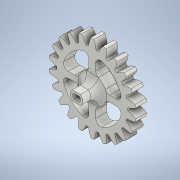
# Autodesk Inventor part: Spur Gear111
Saved by Autodesk Inventor 2021 (Build 250183000, 183)
## iProperties
CustomPartVersion: 1
Created: 2021-02-10
Part Number: Spur Gear111
Material: Steel
Document SubType Name: Modeling
Designer: allen
Categories: <?xml version="1.0" encoding="UTF-16"?> <MemberInstance><Categories><FamilyTemplate><FamilyTemplateParameter ValueType="xs:double" Id="1" ObjectReferenceKey="da_z" ObjectType="kUserParameterObject"/><FamilyTemplateParameter ValueType="xs:double" Id="2" ObjectReferenceKey="da_b" ObjectType="kUserParameterObject"/><FamilyTemplateParameter ValueType="xs:double" Id="3" ObjectReferenceKey="da_beta" ObjectType="kUserParameterObject"/><FamilyTemplateParameter ValueType="xs:double" Id="4" ObjectReferenceKey="da_da" ObjectType="kUserParameterObject"/><FamilyTemplateParameter ValueType="xs:double" Id="5" ObjectReferenceKey="da_aw" ObjectType="kUserParameterObject"/><FamilyTemplateParameter ValueType="xs:string" Id="6" ObjectReferenceKey="EAIAABAAAACIAQAAAAAAAIAAAAAAAAAA" ObjectType="83910656" SubObjectId="SurfaceGeometry"/></FamilyTemplate><ParamToTemplateMap><ParamToTemplate CategoryParameter="//CategoryParameter[@InternalName='046C89C9-8512-4d59-83FE-43B91F4F132A']" TemplateParameter="1"/><ParamToTemplate CategoryParameter="//CategoryParameter[@InternalName='2552DF32-E462-4b46-AEBF-C6C7768E72AC']" TemplateParameter="2"/><ParamToTemplate CategoryParameter="//CategoryParameter[@InternalName='C9EE641D-15FC-4fae-A226-E94C4372FDD7']" TemplateParameter="3"/><ParamToTemplate><ParamToTemplate CategoryParameter="//CategoryParameter[@InternalName='00B6519A-459B-49c7-AD84-2E56D39A5744']" ConstantValue="0.000000"/></ParamToTemplate><ParamToTemplate><ParamToTemplate CategoryParameter="//CategoryParameter[@InternalName='04B31F0E-C7A6-4894-AA32-9629BEFACF47']" ConstantValue="1.000000"/></ParamToTemplate><ParamToTemplate><ParamToTemplate CategoryParameter="//CategoryParameter[@InternalName='43CBEC2E-7847-49e7-A936-2F7889FCB2D9']" ConstantValue="0.250000"/></ParamToTemplate><ParamToTemplate><ParamToTemplate CategoryParameter="//CategoryParameter[@InternalName='B1EFC894-105D-4ebd-86BF-FA20ED196853']" ConstantValue="0.350000"/></ParamToTemplate><ParamToTemplate><ParamToTemplate CategoryParameter="//CategoryParameter[@InternalName='51175063-3D10-4879-93E8-6246FE8B403D']" ConstantValue="2060000000.000000"/></ParamToTemplate><ParamToTemplate><ParamToTemplate CategoryParameter="//CategoryParameter[@InternalName='A3A52E27-4454-46a9-B0BD-C932399B70AF']" ConstantValue="0.300000"/></ParamToTemplate><ParamToTemplate><ParamToTemplate CategoryParameter="//CategoryParameter[@InternalName='91B76062-C214-41d9-B1B9-14D2AB99603D']" ConstantValue="0.225000"/></ParamToTemplate><ParamToTemplate><ParamToTemplate CategoryParameter="//CategoryParameter[@InternalName='374E806E-8B8A-4dda-A9AA-1039D6500AD2']" ConstantValue="4.444444"/></ParamToTemplate><ParamToTemplate><ParamToTemplate CategoryParameter="//CategoryParameter[@InternalName='2D373A89-B862-43d6-8D0B-0CBF12AB9F6C']" ConstantValue="0.349066"/></ParamToTemplate><ParamToTemplate CategoryParameter="//CategoryParameter[@InternalName='37777632-D6A2-4fac-9D53-DB8ACD95C989']" TemplateParameter="4"/><ParamToTemplate CategoryParameter="//CategoryParameter[@InternalName='FD1017F1-B727-4f7e-9707-0F86F1FF9423']" TemplateParameter="5"/><ParamToTemplate><ParamToTemplate CategoryParameter="//CategoryParameter[@InternalName='9E1B4470-B2D3-4ff1-B813-535BB4CDF51A']" ConstantValue="3520000.000000"/></ParamToTemplate><ParamToTemplate><ParamToTemplate CategoryParameter="//CategoryParameter[@InternalName='F8452263-BFF6-458c-9FB1-07C4B99E95CD']" ConstantValue="11400000.000000"/></ParamToTemplate><ParamToTemplate><ParamToTemplate CategoryParameter="//CategoryParameter[@InternalName='3E3BB259-FD49-497f-8171-6EBC954A3479']" ConstantValue="2.000000"/></ParamToTemplate><ParamToTemplate CategoryParameter="//CategoryParameter[@InternalName='27C3BAF2-7550-4e4b-AE2C-0DB134B7D9B7']" TemplateParameter="6"/></ParamToTemplateMap><Category DisplayName="Gear" InternalName="DC85795E-93AB-48d5-8EEE-5A27447B64BD" Mnemonic="Gear"><CategoryParameter DisplayName="z" InternalName="046C89C9-8512-4d59-83FE-43B91F4F132A" Mnemonic="z"/><CategoryParameter DisplayName="b" InternalName="2552DF32-E462-4b46-AEBF-C6C7768E72AC" Mnemonic="b"/><CategoryParameter DisplayName="||b|" InternalName="C9EE641D-15FC-4fae-A226-E94C4372FDD7" Mnemonic="beta"/><CategoryParameter DisplayName="x" InternalName="00B6519A-459B-49c7-AD84-2E56D39A5744" Mnemonic="x"/><CategoryParameter DisplayName="a*" InternalName="04B31F0E-C7A6-4894-AA32-9629BEFACF47" Mnemonic="a"/><CategoryParameter DisplayName="c*" InternalName="43CBEC2E-7847-49e7-A936-2F7889FCB2D9" Mnemonic="c"/><CategoryParameter DisplayName="r|.f|*" InternalName="B1EFC894-105D-4ebd-86BF-FA20ED196853" Mnemonic="rf"/><CategoryParameter DisplayName="E" InternalName="51175063-3D10-4879-93E8-6246FE8B403D" Mnemonic="E"/><CategoryParameter DisplayName="||m|" InternalName="A3A52E27-4454-46a9-B0BD-C932399B70AF" Mnemonic="mi"/><Category DisplayName="SpurGear" InternalName="26C5A22E-A91E-4dfd-A3B3-23CCAFAE1764" Mnemonic="SpurGear"><CategoryParameter DisplayName="m" InternalName="91B76062-C214-41d9-B1B9-14D2AB99603D" Mnemonic="m"/><CategoryParameter DisplayName="P" InternalName="374E806E-8B8A-4dda-A9AA-1039D6500AD2" Mnemonic="PP"/><CategoryParameter DisplayName="||a|" InternalName="2D373A89-B862-43d6-8D0B-0CBF12AB9F6C" Mnemonic="alpha"/><CategoryParameter DisplayName="d|.a|" InternalName="37777632-D6A2-4fac-9D53-DB8ACD95C989" Mnemonic="da"/><CategoryParameter DisplayName="a|.w|" InternalName="FD1017F1-B727-4f7e-9707-0F86F1FF9423" Mnemonic="aw"/><CategoryParameter DisplayName="||s||.Flim|" InternalName="9E1B4470-B2D3-4ff1-B813-535BB4CDF51A" Mnemonic="sFlim"/><CategoryParameter DisplayName="||s||.Hlim|" InternalName="F8452263-BFF6-458c-9FB1-07C4B99E95CD" Mnemonic="sHlim"/><CategoryParameter DisplayName="type" InternalName="3E3BB259-FD49-497f-8171-6EBC954A3479" Mnemonic="type"/><CategoryParameter DisplayName="PitchDiameter" InternalName="27C3BAF2-7550-4e4b-AE2C-0DB134B7D9B7" Mnemonic="IDS_PITCHDIAM"/></Category></Category></Categories></MemberInstance>
Density: 1 g/cm^3
Appearance: Steel
Author: allen
Autodesk Inventor part; units mm, degrees
sketch "Sketch1" plane through (0, 0, 0) normal (0, 0, 1) x (1, 0, 0)
  circle A0 centre (0, 0) radius 27.5
  dimension "d0" = 55
  constraints: 1 centre point
  measures "d0" diameter of A0
extrude "Extrusion1" add sketch "Sketch1" along normal blind 7
ref_plane "Work Plane2" through (0, 0, 3.5) normal (0, 0, 1) x (1, 0, 0)
sketch "Sketch2" plane through (0, 0, 0) normal (0, 0, -1) x (-1, 0, 0)
  circle A0 centre (0, 0) radius 27.5 projected
  circle A1 centre (0, 0) radius 22.5
  dimension "d3" = 45
  constraints: 1 centre point, 1 coincident
  measures "d3" diameter of A1
surface extrude "Pitch Diameter" sketch "Sketch2" against normal through all shown no curves A1
ref_plane "Work Plane8" through (0, 0, 0) normal (0.9898214, 0.1423148, 0) x (0, 0, 1)
ref_plane "Work Plane9" through (0, 0, 0) normal (1, 0, 0) x (0, 1, 0)
spur gear teeth "Spur Gear" teeth 22 pitch diameter 45 tip diameter 55 root diameter 45 face width 10 start plane through (0, 0, 0) normal (0, 0, -1) x (-1, 0, 0)
sketch "Sketch4" plane through (0, 0, 7) normal (0, 0, 1) x (1, 0, 0)
  line L0 (-2.5, 3.1225) -> (2.5, 3.1225)
  line L1 (-2.5, -3.1225) -> (2.5, -3.1225)
  arc A0 (2.5, -3.1225) -> (2.5, 3.1225) centre (0, 0) ccw
  arc A1 (-2.5, 3.1225) -> (-2.5, -3.1225) centre (0, 0) ccw
  dimension "d56" = 4
  dimension "d57" = 4
  dimension "d58" = 5
  dimension "d59" = 5
  constraints: 4 end point, 4 point on circle, 2 centre point, 1 coincident, 1 horizontal, 1 parallel
  measures "d56" radius of A0
  measures "d57" radius of A1
  measures "d58" distance of L0.start L0.end
  measures "d59" distance of L1.start L1.end
extrude "Extrusion3" add sketch "Sketch4" along normal blind 10
sketch "Sketch3" plane through (0, 0, 7) normal (0, 0, 1) x (1, 0, 0)
  line L0 (-1.85, 1.6815) -> (1.85, 1.6815)
  line L1 (-1.85, -1.6815) -> (1.85, -1.6815)
  arc A0 (1.85, -1.6815) -> (1.85, 1.6815) centre (0, 0) ccw
  arc A1 (-1.85, 1.6815) -> (-1.85, -1.6815) centre (0, 0) ccw
  arc A2 (8.793, 1.9193) -> (2.1781, 8.7325) centre (0, 0) ccw
  arc A3 (18.9028, 1.9193) -> (2.1781, 18.8747) centre (0, 0) ccw
  line L2 (2.1781, 18.8747) -> (2.1781, 8.7325)
  line L3 (8.793, 1.9193) -> (18.9028, 1.9193)
  line L4 (0, 0) -> (0, 11.6017)
  line L5 (0, 0) -> (-14.2956, 0)
  arc A4 (-2.1781, 8.7325) -> (-8.793, 1.9193) centre (0, 0) ccw
  arc A5 (-2.1781, 18.8747) -> (-18.9028, 1.9193) centre (0, 0) ccw
  line L6 (-2.1781, 18.8747) -> (-2.1781, 8.7325)
  line L7 (-8.793, 1.9193) -> (-18.9028, 1.9193)
  arc A6 (2.1781, -8.7325) -> (8.793, -1.9193) centre (0, 0) ccw
  arc A7 (2.1781, -18.8747) -> (18.9028, -1.9193) centre (0, 0) ccw
  line L8 (2.1781, -18.8747) -> (2.1781, -8.7325)
  line L9 (8.793, -1.9193) -> (18.9028, -1.9193)
  line L10 (-2.1781, -18.8747) -> (-2.1781, -8.7325)
  arc A8 (-8.793, -1.9193) -> (-2.1781, -8.7325) centre (0, 0) ccw
  arc A9 (-18.9028, -1.9193) -> (-2.1781, -18.8747) centre (0, 0) ccw
  line L11 (-8.793, -1.9193) -> (-18.9028, -1.9193)
  dimension "d49" = 2.5
  dimension "d50" = 2.5
  dimension "d51" = 3.7
  dimension "d52" = 3.7
  dimension "d63" = 19
  dimension "d64" = 9
  dimension "d68" = 10.1423
  dimension "d69" = 10.1098
  constraints: 24 end point, 20 point on circle, 12 symmetric about line, 10 centre point, 6 coincident, 2 horizontal, 2 vertical, 1 parallel, 1 perpendicular, 6 other
  measures "d49" radius of A0
  measures "d50" radius of A1
  measures "d51" distance of L0.start L0.end
  measures "d52" distance of L1.start L1.end
  measures "d63" radius of A3
  measures "d64" radius of A2
  measures "d68" distance of L2.start L2.end
  measures "d69" distance of L3.start L3.end
extrude "Extrusion2" cut sketch "Sketch3" against normal mid plane 100
fillet "Fillet1" radius 5 4 edges at (0, 3.1225, 7) (4, 0, 7) (-4, 0, 7) (0, -3.1225, 7)
fillet "Fillet2" radius 3 16 edges at (2.1781, 8.7325, 3.5) (8.793, 1.9193, 3.5) (8.793, -1.9193, 3.5) (2.1781, -8.7325, 3.5) (2.1781, -18.8747, 3.5) (18.9028, -1.9193, 3.5) (18.9028, 1.9193, 3.5) (2.1781, 18.8747, 3.5) (-2.1781, 18.8747, 3.5) (-2.1781, 8.7325, 3.5) (-18.9028, 1.9193, 3.5) (-8.793, 1.9193, 3.5) (-18.9028, -1.9193, 3.5) (-8.793, -1.9193, 3.5) (-2.1781, -18.8747, 3.5) (-2.1781, -8.7325, 3.5)
equation "\"d0\" = da_da"
equation "\"d3\" = da_d"
equation "\"da_da\" = 55"
equation "\"da_d\" = 45"
body "Solid1"
body "Srf1"
